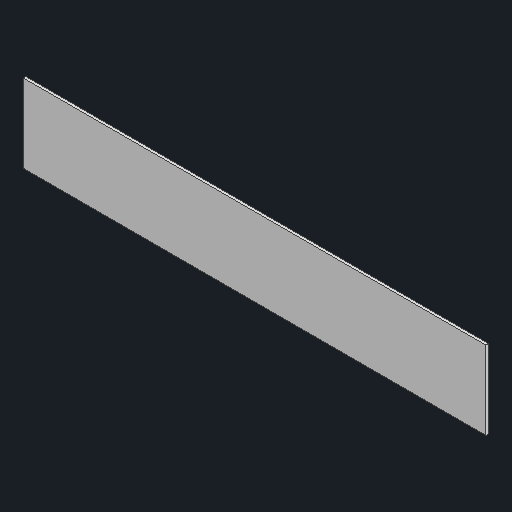
# Autodesk Inventor part: back
Saved by Autodesk Inventor 2023 (Build 270158000, 158)
## iProperties
Created: 2024-04-14
Part Number: back
Material: Generic
Document SubType Name: Modeling
Designer: szymo
Density: 1 g/cm^3
Appearance: Default
Mass: 5.76875 g
Surface Area: 119.575 cm^2
Volume: 5.76875 cm^3
Author: szymo
Autodesk Inventor part; units mm, degrees
ref_plane "YZ Plane" through (0, 0, 0) normal (1, 0, 0) x (0, 1, 0)
ref_plane "XZ Plane" through (0, 0, 0) normal (0, 1, 0) x (-1, 0, 0)
ref_plane "XY Plane" through (0, 0, 0) normal (0, 0, 1) x (1, 0, 0)
sketch "Sketch1" plane through (0, 0, 0) normal (0, 0, 1) x (1, 0, 0)
  line L0 (0, 0) -> (9, 0) projected
  line L1 (9, 0) -> (9, 3) projected
  line L2 (0, 3) -> (9, 3) projected
  line L3 (0, 0) -> (0, 3) projected
  line L4 (-84.5, 30) -> (93.5, 30)
  line L5 (93.5, 30) -> (93.5, 0)
  line L6 (93.5, 0) -> (-84.5, 0)
  line L7 (-84.5, 0) -> (-84.5, 30)
  line L8 (93, -13) -> (93, 32) projected
  point P0 (93, 0)
  point P1 (93, 30)
  dimension "d0" = 178
  dimension "d1" = 84.5
  dimension "d2" = 84.5
  dimension "d4" = 2
  constraints: 8 end point, 2 parallel, 1 collinear, 1 horizontal, 1 perpendicular
  measures "d0" distance of L4.start L4.end
  measures "d1" distance between parallel lines of L1 L5
  measures "d2" distance between parallel lines of L7 L3
  measures "d4" distance from line of L4 L8.end
extrude "Extrusion1" add sketch "Sketch1" along normal blind 1 contours L3 L2 L1 L0 | L6 L7 L4 L8 L1 L2 L3
equation "\"d1\" = d2"
body "Solid1"
